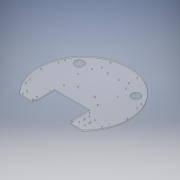
# Autodesk Inventor part: TopPlate
Saved by Autodesk Inventor 2019 (Build 230136000, 136)
## iProperties
Created: 2019-09-28
Part Number: TopPlate
Material: Generic
Document SubType Name: Modeling
Designer: james
Density: 1 g/cm^3
Appearance: Polycarbonate - Clear
Mass: 617.456 g
Surface Area: 2657.72 cm^2
Volume: 617.456 cm^3
Author: james
Autodesk Inventor part; units mm, degrees
ref_plane "YZ Plane" through (0, 0, 0) normal (1, 0, 0) x (0, 1, 0)
ref_plane "XZ Plane" through (0, 0, 0) normal (0, 1, 0) x (-1, 0, 0)
ref_plane "XY Plane" through (0, 0, 0) normal (0, 0, 1) x (1, 0, 0)
sketch "Sketch1" plane through (0, 0, 0) normal (0, 1, 0) x (-1, 0, 0)
  circle A0 centre (0, 0) radius 203.2
  dimension "d0" = 406.4
  constraints: 1 centre point, 1 coincident
  measures "d0" diameter of A0
extrude "Extrusion1" add sketch "Sketch1" along normal blind 4.7625
sketch "Sketch2" plane through (0, 4.7625, 0) normal (0, 1, 0) x (1, 0, 0)
  point P0 (0, 0)
  point P1 (-88.9, 64)
  point P2 (-176.9, 64)
  point P3 (-88.9, -64)
  point P4 (-176.9, -64)
  dimension "d3" = 0
  dimension "d4" = 0
  dimension "d5" = 0
  dimension "d6" = 0
  dimension "d7" = 128
  dimension "d8" = 88
  dimension "d9" = 64
  dimension "d10" = 88.9
  measures "d3" horizontal distance of point (-176.9, -64) point (-176.9, 64)
  measures "d4" horizontal distance of point (-88.9, -64) point (-88.9, 64)
  measures "d5" vertical distance of point (-176.9, -64) point (-88.9, -64)
  measures "d6" vertical distance of point (-176.9, 64) point (-88.9, 64)
  measures "d7" distance of point (-176.9, -64) point (-176.9, 64)
  measures "d8" distance of point (-176.9, -64) point (-88.9, -64)
  measures "d9" vertical distance of point (-88.9, -64) point (0, 0)
  measures "d10" horizontal distance of point (-88.9, 64) point (0, 0)
hole "Hole1" at (-88.9, 4.7625, -64) at (-176.9, 4.7625, -64) at (-88.9, 4.7625, 64) at (-176.9, 4.7625, 64) direction (0, -1, 0) diameter 3.2766 end through all clearance for "Flat Head Machine Screw (82)" size "#4" standard "Ansi Unified Screw Threads"
sketch "Sketch3" plane through (0, 4.7625, 0) normal (0, 1, 0) x (1, 0, 0)
  point P0 (0, 0)
  point P1 (88.9, 64)
  point P2 (176.9, 64)
  point P3 (88.9, -62)
  point P4 (176.9, -62)
  dimension "d18" = 0
  dimension "d19" = 0
  dimension "d20" = 0
  dimension "d21" = 0
  dimension "d22" = 126
  dimension "d23" = 88
  dimension "d24" = 64
  dimension "d25" = 88.9
  measures "d18" horizontal distance of point (176.9, -62) point (176.9, 64)
  measures "d19" vertical distance of point (88.9, 64) point (176.9, 64)
  measures "d20" vertical distance of point (88.9, -62) point (176.9, -62)
  measures "d21" horizontal distance of point (88.9, 64) point (88.9, -62)
  measures "d22" distance of point (176.9, -62) point (176.9, 64)
  measures "d23" distance of point (88.9, -62) point (176.9, -62)
  measures "d24" vertical distance of point (0, 0) point (88.9, 64)
  measures "d25" horizontal distance of point (0, 0) point (88.9, -62)
hole "Hole2" at (88.9, 4.7625, -64) at (176.9, 4.7625, -64) at (88.9, 4.7625, 62) at (176.9, 4.7625, 62) direction (0, -1, 0) diameter 3.2766 end through all clearance for "Flat Head Machine Screw (82)" size "#4" standard "Ansi Unified Screw Threads"
sketch "Sketch4" plane through (0, 4.7625, 0) normal (0, 1, 0) x (1, 0, 0)
  point P0 (0, 0)
  point P1 (-38.1, 12.7)
  point P2 (38.1, 12.7)
  dimension "d33" = 38.1
  dimension "d34" = 0
  dimension "d35" = 76.2
  dimension "d125" = 12.7
  measures "d33" horizontal distance of point (-38.1, 12.7) point (0, 0)
  measures "d34" vertical distance of point (38.1, 12.7) point (-38.1, 12.7)
  measures "d35" distance of point (-38.1, 12.7) point (38.1, 12.7)
  measures "d125" vertical distance of point (-38.1, 12.7) point (0, 0)
hole "Hole3" at (-38.1, 4.7625, -12.7) at (38.1, 4.7625, -12.7) direction (0, -1, 0) diameter 5.1054 end through all clearance for "Flat Head Machine Screw (82)" size "#10" standard "Ansi Unified Screw Threads"
sketch "Sketch5" plane through (0, 4.7625, 0) normal (0, 1, 0) x (1, 0, 0)
  line L0 (-79.375, -50.8) -> (79.375, -50.8)
  line L1 (79.375, -50.8) -> (79.375, -418.3154)
  line L2 (79.375, -418.3154) -> (-79.375, -418.3154)
  line L3 (-79.375, -418.3154) -> (-79.375, -50.8)
  point P0 (0, 0)
  dimension "d44" = 158.75
  dimension "d45" = 79.375
  dimension "d46" = 50.8
  constraints: 8 end point, 2 parallel, 1 horizontal, 1 perpendicular
  measures "d44" distance of L1.end L2.end
  measures "d45" distance from line of L3 point (0, 0)
  measures "d46" distance from line of L0 point (0, 0)
extrude "Extrusion2" cut sketch "Sketch5" against normal blind 25.4
sketch "Sketch6" plane through (0, 4.7625, 0) normal (0, 1, 0) x (1, 0, 0)
  line L0 (-85.725, -133.35) -> (85.725, -133.35)
  line L1 (85.725, -133.35) -> (85.725, -214.7916)
  line L2 (85.725, -214.7916) -> (-85.725, -214.7916)
  line L3 (-85.725, -214.7916) -> (-85.725, -133.35)
  line L4 (-79.375, -50.8) -> (79.375, -50.8) projected
  line L5 (-79.375, -187.0557) -> (-79.375, -50.8) projected
  line L6 (79.375, -50.8) -> (79.375, -187.0557) projected
  point P0 (0, 0)
  dimension "d49" = 82.55
  dimension "d50" = 6.35
  dimension "d51" = 6.35
  constraints: 8 end point, 2 parallel, 1 horizontal, 1 perpendicular
  measures "d49" distance between parallel lines of L0 L4
  measures "d50" distance between parallel lines of L3 L5
  measures "d51" distance between parallel lines of L6 L1
extrude "Extrusion3" cut sketch "Sketch6" against normal blind 25.4 contours L0 L1 L2 L3
sketch "Sketch8" plane through (0, 4.7625, 0) normal (0, 1, 0) x (1, 0, 0)
  line L0 (-85.725, -133.35) -> (-79.375, -133.35) projected
  line L1 (-85.725, -184.2321) -> (-85.725, -133.35) projected
  point P0 (0, 0)
  point P1 (-136.525, -118.11)
  point P2 (-92.075, -118.11)
  point P3 (-136.525, -137.16)
  point P4 (-92.075, -137.16)
  dimension "d65" = 0
  dimension "d66" = 0
  dimension "d67" = 0
  dimension "d68" = 44.45
  dimension "d69" = 19.05
  dimension "d70" = 0
  dimension "d71" = 15.24
  dimension "d72" = 6.35
  measures "d65" horizontal distance of point (-92.075, -137.16) point (-92.075, -118.11)
  measures "d66" horizontal distance of point (-136.525, -118.11) point (-136.525, -137.16)
  measures "d67" vertical distance of point (-92.075, -118.11) point (-136.525, -118.11)
  measures "d68" distance of point (-92.075, -118.11) point (-136.525, -118.11)
  measures "d69" distance of point (-136.525, -137.16) point (-136.525, -118.11)
  measures "d70" vertical distance of point (-92.075, -137.16) point (-136.525, -137.16)
  measures "d71" distance from line of L0 point (-92.075, -118.11)
  measures "d72" distance from line of L1 point (-92.075, -118.11)
hole "Hole5" at (-136.525, 4.7625, 118.11) at (-92.075, 4.7625, 118.11) at (-136.525, 4.7625, 137.16) at (-92.075, 4.7625, 137.16) direction (0, -1, 0) diameter 4.4958 end through all clearance for "Flat Head Machine Screw (82)" size "#8" standard "Ansi Unified Screw Threads"
sketch "Sketch9" plane through (0, 4.7625, 0) normal (0, 1, 0) x (1, 0, 0)
  point P0 (0, 0)
  point P1 (-190.5, 0)
  point P2 (-171.45, 88.9)
  point P3 (-171.45, -88.9)
  dimension "d80" = 190.5
  dimension "d81" = 171.45
  dimension "d82" = 88.9
  dimension "d83" = 88.9
  dimension "d84" = 171.45
  measures "d80" distance of point (-190.5, 0) point (0, 0)
  measures "d81" horizontal distance of point (-171.45, 88.9) point (0, 0)
  measures "d82" vertical distance of point (0, 0) point (-171.45, 88.9)
  measures "d83" vertical distance of point (-171.45, -88.9) point (0, 0)
  measures "d84" horizontal distance of point (0, 0) point (-171.45, -88.9)
hole "Hole6" at (-190.5, 4.7625, 0) at (-171.45, 4.7625, -88.9) at (-171.45, 4.7625, 88.9) direction (0, -1, 0) diameter 4.4958 end through all clearance for "Flat Head Machine Screw (82)" size "#8" standard "Ansi Unified Screw Threads"
sketch "Sketch10" plane through (0, 4.7625, 0) normal (0, 1, 0) x (1, 0, 0)
  point P0 (0, 0)
  point P1 (196.85, 0)
  point P2 (171.45, 88.9)
  point P3 (171.45, -88.9)
  dimension "d92" = 0
  dimension "d93" = 196.85
  dimension "d94" = 171.45
  dimension "d95" = 171.45
  dimension "d96" = 88.9
  dimension "d97" = 88.9
  measures "d92" vertical distance of point (196.85, 0) point (0, 0)
  measures "d93" distance of point (0, 0) point (196.85, 0)
  measures "d94" horizontal distance of point (0, 0) point (171.45, 88.9)
  measures "d95" horizontal distance of point (0, 0) point (171.45, -88.9)
  measures "d96" vertical distance of point (0, 0) point (171.45, -88.9)
  measures "d97" vertical distance of point (0, 0) point (171.45, 88.9)
hole "Hole7" at (196.85, 4.7625, 0) at (171.45, 4.7625, -88.9) at (171.45, 4.7625, 88.9) direction (0, -1, 0) diameter 4.4958 end through all clearance for "Flat Head Machine Screw (82)" size "#8" standard "Ansi Unified Screw Threads"
sketch "Sketch11" plane through (0, 4.7625, 0) normal (0, 1, 0) x (1, 0, 0)
  line L0 (-153.6895, -146.05) -> (154.4346, -146.05)
  line L1 (154.4346, -146.05) -> (154.4346, -205.4298)
  line L2 (154.4346, -205.4298) -> (-153.6895, -205.4298)
  line L3 (-153.6895, -205.4298) -> (-153.6895, -146.05)
  line L4 (-79.375, -50.8) -> (79.375, -50.8) projected
  point P0 (0, 0)
  dimension "d105" = 95.25
  constraints: 8 end point, 2 parallel, 1 horizontal, 1 perpendicular
  measures "d105" distance between parallel lines of L0 L4
extrude "Extrusion4" cut sketch "Sketch11" against normal blind 25.4
sketch "Sketch12" plane through (0, 4.7625, 0) normal (0, 1, 0) x (1, 0, 0)
  point P0 (0, 0)
  point P1 (-76.2, 114.3)
  point P2 (-76.2, -12.7)
  point P3 (76.2, 114.3)
  point P4 (76.2, -12.7)
  dimension "d108" = 0
  dimension "d109" = 0
  dimension "d110" = 0
  dimension "d111" = 0
  dimension "d112" = 76.2
  dimension "d113" = 76.2
  dimension "d115" = 127
  dimension "d123" = 12.7
  measures "d108" vertical distance of point (76.2, -12.7) point (-76.2, -12.7)
  measures "d109" vertical distance of point (76.2, 114.3) point (-76.2, 114.3)
  measures "d110" horizontal distance of point (76.2, -12.7) point (76.2, 114.3)
  measures "d111" horizontal distance of point (-76.2, 114.3) point (-76.2, -12.7)
  measures "d112" horizontal distance of point (0, 0) point (-76.2, -12.7)
  measures "d113" horizontal distance of point (0, 0) point (76.2, -12.7)
  measures "d115" distance of point (76.2, 114.3) point (76.2, -12.7)
  measures "d123" vertical distance of point (76.2, -12.7) point (0, 0)
hole "Hole8" at (-76.2, 4.7625, -114.3) at (-76.2, 4.7625, 12.7) at (76.2, 4.7625, -114.3) at (76.2, 4.7625, 12.7) direction (0, -1, 0) diameter 4.4958 end through all clearance for "Flat Head Machine Screw (82)" size "#8" standard "Ansi Unified Screw Threads"
sketch "Sketch13" plane through (0, 4.7625, 0) normal (0, 1, 0) x (1, 0, 0)
  circle A0 centre (-38.1, 12.7) radius 2.5527 projected
  point P0 (0, 0)
  point P1 (-25.4, 133.35)
  point P2 (25.4, 133.35)
  dimension "d127" = 0
  dimension "d128" = 50.8
  dimension "d129" = 12.7
  dimension "d137" = 120.65
  measures "d127" vertical distance of point (-25.4, 133.35) point (25.4, 133.35)
  measures "d128" distance of point (25.4, 133.35) point (-25.4, 133.35)
  measures "d129" horizontal distance of A0.centre point (-25.4, 133.35)
  measures "d137" vertical distance of point (-25.4, 133.35) A0.centre
hole "Hole9" at (-25.4, 4.7625, -133.35) at (25.4, 4.7625, -133.35) direction (0, -1, 0) diameter 4.4958 end through all clearance for "Flat Head Machine Screw (82)" size "#8" standard "Ansi Unified Screw Threads"
sketch "Sketch14" plane through (0, 4.7625, 0) normal (0, 1, 0) x (1, 0, 0)
  circle A0 centre (-127, 107.95) radius 19.05
  circle A1 centre (127, 107.95) radius 19.05
  point P0 (0, 0)
  dimension "d138" = 38.1
  dimension "d139" = 127
  dimension "d140" = 107.95
  dimension "d141" = 38.1
  dimension "d142" = 0
  dimension "d143" = 127
  constraints: 2 centre point
  measures "d138" diameter of A0
  measures "d139" horizontal distance of A0.centre point (0, 0)
  measures "d140" vertical distance of point (0, 0) A0.centre
  measures "d141" diameter of A1
  measures "d142" vertical distance of A1.centre A0.centre
  measures "d143" horizontal distance of point (0, 0) A1.centre
extrude "Extrusion5" cut sketch "Sketch14" against normal blind 25.4
sketch "Sketch15" plane through (0, 4.7625, 0) normal (0, 1, 0) x (1, 0, 0)
  arc A0 (141.2786, -146.05) -> (-141.2786, -146.05) centre (0, 0) ccw projected
  point P0 (101.6, -76.2)
  point P1 (101.6, -95.25)
  point P2 (101.6, -101.6)
  point P3 (101.6, -120.65)
  point P4 (127, -120.65)
  point P5 (127, -101.6)
  point P6 (127, -95.25)
  point P7 (127, -76.2)
  dimension "d146" = 0
  dimension "d147" = 0
  dimension "d148" = 0
  dimension "d149" = 0
  dimension "d150" = 0
  dimension "d151" = 19.05
  dimension "d152" = 19.05
  dimension "d153" = 6.35
  dimension "d154" = 0
  dimension "d155" = 0
  dimension "d156" = 0
  dimension "d157" = 0
  dimension "d158" = 25.4
  dimension "d159" = 0
  dimension "d160" = 101.6
  dimension "d161" = 76.2
  measures "d146" vertical distance of point (127, -76.2) point (101.6, -76.2)
  measures "d147" vertical distance of point (101.6, -95.25) point (127, -95.25)
  measures "d148" horizontal distance of point (127, -95.25) point (127, -76.2)
  measures "d149" horizontal distance of point (127, -101.6) point (127, -95.25)
  measures "d150" horizontal distance of point (127, -101.6) point (127, -120.65)
  measures "d151" distance of point (127, -101.6) point (127, -120.65)
  measures "d152" distance of point (127, -76.2) point (127, -95.25)
  measures "d153" distance of point (127, -101.6) point (127, -95.25)
  measures "d154" vertical distance of point (127, -101.6) point (101.6, -101.6)
  measures "d155" vertical distance of point (127, -120.65) point (101.6, -120.65)
  measures "d156" horizontal distance of point (101.6, -95.25) point (101.6, -101.6)
  measures "d157" horizontal distance of point (101.6, -101.6) point (101.6, -120.65)
  measures "d158" distance of point (127, -120.65) point (101.6, -120.65)
  measures "d159" horizontal distance of point (101.6, -76.2) point (101.6, -95.25)
  measures "d160" horizontal distance of point (101.6, -76.2) point (0, 0)
  measures "d161" vertical distance of point (101.6, -76.2) point (0, 0)
hole "Hole10" at (101.6, 4.7625, 76.2) at (101.6, 4.7625, 95.25) at (101.6, 4.7625, 101.6) at (101.6, 4.7625, 120.65) at (127, 4.7625, 120.65) at (127, 4.7625, 101.6) at (127, 4.7625, 95.25) at (127, 4.7625, 76.2) direction (0, -1, 0) diameter 3.81 end through all clearance for "Flat Head Machine Screw (82)" size "#6" standard "Ansi Unified Screw Threads"
sketch "Sketch16" plane through (0, 4.7625, 0) normal (0, 1, 0) x (1, 0, 0)
  point P0 (0, 0)
  point P1 (-60.325, 142.875)
  point P2 (-60.325, 180.975)
  point P3 (60.325, 142.875)
  point P4 (60.325, 180.975)
  dimension "d169" = 38.1
  dimension "d170" = 142.875
  dimension "d171" = 60.325
  dimension "d172" = 0
  dimension "d173" = 0
  dimension "d174" = 0
  dimension "d175" = 0
  dimension "d176" = 60.325
  measures "d169" distance of point (-60.325, 142.875) point (-60.325, 180.975)
  measures "d170" vertical distance of point (0, 0) point (-60.325, 142.875)
  measures "d171" horizontal distance of point (0, 0) point (-60.325, 142.875)
  measures "d172" horizontal distance of point (-60.325, 142.875) point (-60.325, 180.975)
  measures "d173" horizontal distance of point (60.325, 180.975) point (60.325, 142.875)
  measures "d174" vertical distance of point (-60.325, 180.975) point (60.325, 180.975)
  measures "d175" vertical distance of point (-60.325, 142.875) point (60.325, 142.875)
  measures "d176" horizontal distance of point (0, 0) point (60.325, 142.875)
hole "Hole11" at (-60.325, 4.7625, -142.875) at (-60.325, 4.7625, -180.975) at (60.325, 4.7625, -142.875) at (60.325, 4.7625, -180.975) direction (0, -1, 0) diameter 4.4958 end through all clearance for "Flat Head Machine Screw (82)" size "#8" standard "Ansi Unified Screw Threads"
body "Solid1"
